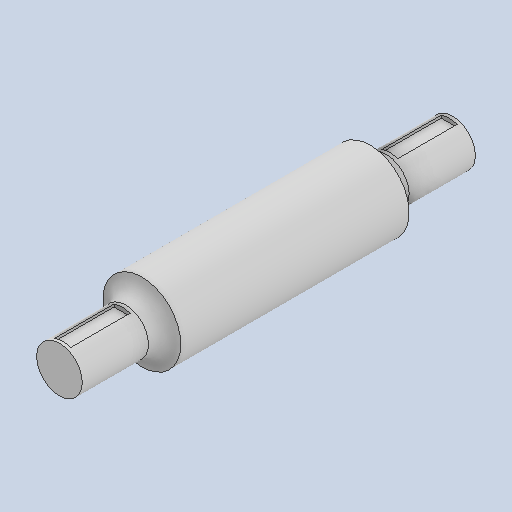
# Autodesk Inventor part: Eje cuñero
Saved by Autodesk Inventor 2022 (Build 260153000, 153)
## iProperties
Created: 2024-04-07
Part Number: Eje cuñero
Material: Genérico
Document SubType Name: Modeling
Designer: Lourdes Ac Minera
Density: 1 g/cm^3
Appearance: Valor por defecto
Author: Lourdes Ac Minera
Autodesk Inventor part; units mm, degrees
ref_plane "YZ Plane" through (0, 0, 0) normal (1, 0, 0) x (0, 1, 0)
ref_plane "XY Plane" through (0, 0, 0) normal (0, 0, 1) x (1, 0, 0)
sketch "Boceto1" plane through (0, 0, 0) normal (0, 0, 1) x (1, 0, 0)
  circle A0 centre (0, 0) radius 17.07
  dimension "d0" = 34.14
  constraints: 1 centre point, 1 coincident
  measures "d0" diameter of A0
extrude "Extrusión1" add sketch "Boceto1" along normal blind 100
sketch "Boceto2" plane through (0, 0, 100) normal (0, 0, 1) x (1, 0, 0)
  circle A0 centre (0, 0) radius 10
  dimension "d3" = 20
  constraints: 1 centre point, 1 coincident
  measures "d3" diameter of A0
extrude "Extrusión2" add sketch "Boceto2" along normal blind 36.08
sketch "Boceto3" plane through (0, 0, 0) normal (0, 0, -1) x (-1, 0, 0)
  circle A0 centre (0, 0) radius 10
  dimension "d6" = 20
  constraints: 1 centre point, 1 coincident
  measures "d6" diameter of A0
extrude "Extrusión3" add sketch "Boceto3" along normal blind 36.08
fillet "Empalme1" radius 7.07 1 edges at (-10, 0, 100)
fillet "Empalme2" radius 7.07 1 edges at (10, 0, 0)
ref_plane "Plano de trabajo1" through (0, 10, 100) normal (0, 1, 0) x (-1, 0, 0)
sketch "Boceto4" plane through (0, 10, 100) normal (0, 1, 0) x (-1, 0, 0)
  line L0 (10, 36.08) -> (-10, 36.08) projected
  line L1 (-3.5, 34.6498) -> (3.5, 34.6498)
  line L2 (3.5, 34.6498) -> (3.5, 8.6498)
  line L3 (3.5, 8.6498) -> (-3.5, 8.6498)
  line L4 (-3.5, 8.6498) -> (-3.5, 34.6498)
  line L5 (-3.5, 34.6498) -> (3.5, 8.6498) construction
  line L6 (3.5, 34.6498) -> (-3.5, 8.6498) construction
  line L7 (10, -107.07) -> (-10, -107.07) projected
  line L8 (-10, -136.08) -> (10, -136.08) projected
  line L9 (10, -107.07) -> (10, -136.08) projected
  line L10 (-3.5, -108.575) -> (3.5, -108.575)
  line L11 (3.5, -108.575) -> (3.5, -134.575)
  line L12 (3.5, -134.575) -> (-3.5, -134.575)
  line L13 (-3.5, -134.575) -> (-3.5, -108.575)
  point P0 (0, -100)
  point P1 (0, 21.6498)
  dimension "d11" = 7
  dimension "d12" = 26
  dimension "d13" = 7
  dimension "d14" = 26
  constraints: 20 end point, 4 parallel, 2 horizontal, 2 midpoint, 2 perpendicular
  measures "d11" distance of L2.end L3.end
  measures "d12" distance of L1.end L2.end
  measures "d13" distance of L11.end L13.start
  measures "d14" distance of L11.start L11.end
extrude "Extrusión4" cut sketch "Boceto4" against normal blind 1.77
